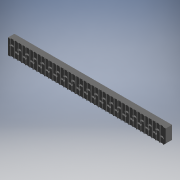
# Autodesk Inventor part: IDSD-20_ub
Saved by Autodesk Inventor 2017.3 (Build 213256000, 256)
## iProperties
Part Number: IDSD-20_ub
Material: Generic
Catalog Web Link: www.cadenas.de
Description: IDSS, IDSD Series - Upper Body-.100" Slim Body, IDC Ribbon Cable Assembly, Socket
Vendor: SAMTEC
Document SubType Name: Modeling
Designer: partserver
Manufacturer: SAMTEC
Mass: 0.43638 g
Surface Area: 11.6206 cm^2
Volume: 0.43638 cm^3
Density: 1 g/cm^3
Appearance: PSOLRGB-127-127-127
Category: PARTsolutions
Company: SAMTEC
Title: IDSD-20_ub
Author: Cadenas PARTsolutions
Comments: .100" Slim Body, IDC Ribbon Cable Assembly, Socket
PSOL_IDENT_0: {$CADENAS_DATA\23d-libs\samtec\modelling\idsd\parts\idsd_upper_body.prj},187 {VTYP=3D},{NB=IDSD-20_u
PSOL_IDENT_1: b},{LINA=IDSD-20_ub},{NN=IDSS, IDSD Series - Upper Body},{DATE=12.08.2019 09:04:52},{GEOMDATE=14.12.
PSOL_IDENT_2: 2015 10:21:00},{VERSION=},{LINEID=20},{WBVAR=POS},{WBNUMERIC=}  {NB=IDSD-20_ub},{LINA=IDSD-20_ub},{K
PSOL_IDENT_3: T=DUMMY},{PN=IDSD-20},{SERIES=IDSD},{POS=20},{POSNO=20},{A=2.05900000},{B=0.20},{C=0.10},{D=0.365}
NB: IDSD-20_ub
NN: IDSS, IDSD Series - Upper Body
NT: .100" Slim Body, IDC Ribbon Cable Assembly, Socket
NBSYN: $PN._ub
LINA: IDSD-20_ub
CATALOG: Samtec
SERIES: IDSD
POS: -20
B: 0.2
C: 0.1
SUPPLIER: SAMTEC
ARTICLENO: IDSD-20_ub
BOMINFO: IDSD-20_ub
CREATOR: CADENAS GmbH
Autodesk Inventor part; units mm, degrees
sketch "Sketch_1" plane through (0, 0, 0) normal (0, 1, 0) x (-1, 0, 0)
  line L0 (26.1493, 1.778) -> (25.3873, 2.54)
  line L1 (25.3873, 2.54) -> (-26.1493, 2.54)
  line L2 (-26.1493, 2.54) -> (-26.1493, -2.54)
  line L3 (-26.1493, -2.54) -> (26.1493, -2.54)
  line L4 (26.1493, -2.54) -> (26.1493, 1.778)
  line L5 (-24.2126, -0.9144) -> (-24.2126, -0.4064)
  line L6 (-24.2126, -0.4064) -> (-25.5461, -0.4064)
  line L7 (-25.5461, -0.4064) -> (-25.5461, -0.9144)
  line L8 (-25.5461, -0.9144) -> (-24.2126, -0.9144)
  line L9 (-22.714, 0.4064) -> (-22.714, 0.9144)
  line L10 (-22.714, 0.9144) -> (-24.0475, 0.9144)
  line L11 (-24.0475, 0.9144) -> (-24.0475, 0.4064)
  line L12 (-24.0475, 0.4064) -> (-22.714, 0.4064)
  line L13 (-21.6726, -0.9144) -> (-21.6726, -0.4064)
  line L14 (-21.6726, -0.4064) -> (-23.0061, -0.4064)
  line L15 (-23.0061, -0.4064) -> (-23.0061, -0.9144)
  line L16 (-23.0061, -0.9144) -> (-21.6726, -0.9144)
  line L17 (-20.174, 0.4064) -> (-20.174, 0.9144)
  line L18 (-20.174, 0.9144) -> (-21.5075, 0.9144)
  line L19 (-21.5075, 0.9144) -> (-21.5075, 0.4064)
  line L20 (-21.5075, 0.4064) -> (-20.174, 0.4064)
  line L21 (-19.1325, -0.9144) -> (-19.1325, -0.4064)
  line L22 (-19.1325, -0.4064) -> (-20.466, -0.4064)
  line L23 (-20.466, -0.4064) -> (-20.466, -0.9144)
  line L24 (-20.466, -0.9144) -> (-19.1325, -0.9144)
  line L25 (-17.6339, 0.4064) -> (-17.6339, 0.9144)
  line L26 (-17.6339, 0.9144) -> (-18.9674, 0.9144)
  line L27 (-18.9674, 0.9144) -> (-18.9674, 0.4064)
  line L28 (-18.9674, 0.4064) -> (-17.6339, 0.4064)
  line L29 (-16.5925, -0.9144) -> (-16.5925, -0.4064)
  line L30 (-16.5925, -0.4064) -> (-17.9261, -0.4064)
  line L31 (-17.9261, -0.4064) -> (-17.9261, -0.9144)
  line L32 (-17.9261, -0.9144) -> (-16.5925, -0.9144)
  line L33 (-15.0939, 0.4064) -> (-15.0939, 0.9144)
  line L34 (-15.0939, 0.9144) -> (-16.4275, 0.9144)
  line L35 (-16.4275, 0.9144) -> (-16.4275, 0.4064)
  line L36 (-16.4275, 0.4064) -> (-15.0939, 0.4064)
  line L37 (-14.0526, -0.9144) -> (-14.0526, -0.4064)
  line L38 (-14.0526, -0.4064) -> (-15.3861, -0.4064)
  line L39 (-15.3861, -0.4064) -> (-15.3861, -0.9144)
  line L40 (-15.3861, -0.9144) -> (-14.0526, -0.9144)
  line L41 (-12.554, 0.4064) -> (-12.554, 0.9144)
  line L42 (-12.554, 0.9144) -> (-13.8874, 0.9144)
  line L43 (-13.8874, 0.9144) -> (-13.8874, 0.4064)
  line L44 (-13.8874, 0.4064) -> (-12.554, 0.4064)
  line L45 (-11.5125, -0.9144) -> (-11.5125, -0.4064)
  line L46 (-11.5125, -0.4064) -> (-12.846, -0.4064)
  line L47 (-12.846, -0.4064) -> (-12.846, -0.9144)
  line L48 (-12.846, -0.9144) -> (-11.5125, -0.9144)
  line L49 (-10.014, 0.4064) -> (-10.014, 0.9144)
  line L50 (-10.014, 0.9144) -> (-11.3474, 0.9144)
  line L51 (-11.3474, 0.9144) -> (-11.3474, 0.4064)
  line L52 (-11.3474, 0.4064) -> (-10.014, 0.4064)
  line L53 (-8.9726, -0.9144) -> (-8.9726, -0.4064)
  line L54 (-8.9726, -0.4064) -> (-10.306, -0.4064)
  line L55 (-10.306, -0.4064) -> (-10.306, -0.9144)
  line L56 (-10.306, -0.9144) -> (-8.9726, -0.9144)
  line L57 (-7.474, 0.4064) -> (-7.474, 0.9144)
  line L58 (-7.474, 0.9144) -> (-8.8074, 0.9144)
  line L59 (-8.8074, 0.9144) -> (-8.8074, 0.4064)
  line L60 (-8.8074, 0.4064) -> (-7.474, 0.4064)
  line L61 (-6.4325, -0.9144) -> (-6.4325, -0.4064)
  line L62 (-6.4325, -0.4064) -> (-7.7661, -0.4064)
  line L63 (-7.7661, -0.4064) -> (-7.7661, -0.9144)
  line L64 (-7.7661, -0.9144) -> (-6.4325, -0.9144)
  line L65 (-4.934, 0.4064) -> (-4.934, 0.9144)
  line L66 (-4.934, 0.9144) -> (-6.2675, 0.9144)
  line L67 (-6.2675, 0.9144) -> (-6.2675, 0.4064)
  line L68 (-6.2675, 0.4064) -> (-4.934, 0.4064)
  line L69 (-3.8925, -0.9144) -> (-3.8925, -0.4064)
  line L70 (-3.8925, -0.4064) -> (-5.226, -0.4064)
  line L71 (-5.226, -0.4064) -> (-5.226, -0.9144)
  line L72 (-5.226, -0.9144) -> (-3.8925, -0.9144)
  line L73 (-2.3939, 0.4064) -> (-2.3939, 0.9144)
  line L74 (-2.3939, 0.9144) -> (-3.7275, 0.9144)
  line L75 (-3.7275, 0.9144) -> (-3.7275, 0.4064)
  line L76 (-3.7275, 0.4064) -> (-2.3939, 0.4064)
  line L77 (-1.3525, -0.9144) -> (-1.3525, -0.4064)
  line L78 (-1.3525, -0.4064) -> (-2.686, -0.4064)
  line L79 (-2.686, -0.4064) -> (-2.686, -0.9144)
  line L80 (-2.686, -0.9144) -> (-1.3525, -0.9144)
  line L81 (0.1461, 0.4064) -> (0.1461, 0.9144)
  line L82 (0.1461, 0.9144) -> (-1.1875, 0.9144)
  line L83 (-1.1875, 0.9144) -> (-1.1875, 0.4064)
  line L84 (-1.1875, 0.4064) -> (0.1461, 0.4064)
  line L85 (1.1875, -0.9144) -> (1.1875, -0.4064)
  line L86 (1.1875, -0.4064) -> (-0.146, -0.4064)
  line L87 (-0.146, -0.4064) -> (-0.146, -0.9144)
  line L88 (-0.146, -0.9144) -> (1.1875, -0.9144)
  line L89 (2.686, 0.4064) -> (2.686, 0.9144)
  line L90 (2.686, 0.9144) -> (1.3525, 0.9144)
  line L91 (1.3525, 0.9144) -> (1.3525, 0.4064)
  line L92 (1.3525, 0.4064) -> (2.686, 0.4064)
  line L93 (3.7275, -0.9144) -> (3.7275, -0.4064)
  line L94 (3.7275, -0.4064) -> (2.3939, -0.4064)
  line L95 (2.3939, -0.4064) -> (2.3939, -0.9144)
  line L96 (2.3939, -0.9144) -> (3.7275, -0.9144)
  line L97 (5.226, 0.4064) -> (5.226, 0.9144)
  line L98 (5.226, 0.9144) -> (3.8925, 0.9144)
  line L99 (3.8925, 0.9144) -> (3.8925, 0.4064)
  line L100 (3.8925, 0.4064) -> (5.226, 0.4064)
  line L101 (6.2675, -0.9144) -> (6.2675, -0.4064)
  line L102 (6.2675, -0.4064) -> (4.934, -0.4064)
  line L103 (4.934, -0.4064) -> (4.934, -0.9144)
  line L104 (4.934, -0.9144) -> (6.2675, -0.9144)
  line L105 (7.7661, 0.4064) -> (7.7661, 0.9144)
  line L106 (7.7661, 0.9144) -> (6.4325, 0.9144)
  line L107 (6.4325, 0.9144) -> (6.4325, 0.4064)
  line L108 (6.4325, 0.4064) -> (7.7661, 0.4064)
  line L109 (8.8074, -0.9144) -> (8.8074, -0.4064)
  line L110 (8.8074, -0.4064) -> (7.474, -0.4064)
  line L111 (7.474, -0.4064) -> (7.474, -0.9144)
  line L112 (7.474, -0.9144) -> (8.8074, -0.9144)
  line L113 (10.306, 0.4064) -> (10.306, 0.9144)
  line L114 (10.306, 0.9144) -> (8.9726, 0.9144)
  line L115 (8.9726, 0.9144) -> (8.9726, 0.4064)
  line L116 (8.9726, 0.4064) -> (10.306, 0.4064)
  line L117 (11.3474, -0.9144) -> (11.3474, -0.4064)
  line L118 (11.3474, -0.4064) -> (10.014, -0.4064)
  line L119 (10.014, -0.4064) -> (10.014, -0.9144)
  line L120 (10.014, -0.9144) -> (11.3474, -0.9144)
  line L121 (12.846, 0.4064) -> (12.846, 0.9144)
  line L122 (12.846, 0.9144) -> (11.5125, 0.9144)
  line L123 (11.5125, 0.9144) -> (11.5125, 0.4064)
  line L124 (11.5125, 0.4064) -> (12.846, 0.4064)
  line L125 (13.8874, -0.9144) -> (13.8874, -0.4064)
  line L126 (13.8874, -0.4064) -> (12.554, -0.4064)
  line L127 (12.554, -0.4064) -> (12.554, -0.9144)
  line L128 (12.554, -0.9144) -> (13.8874, -0.9144)
  line L129 (15.3861, 0.4064) -> (15.3861, 0.9144)
  line L130 (15.3861, 0.9144) -> (14.0526, 0.9144)
  line L131 (14.0526, 0.9144) -> (14.0526, 0.4064)
  line L132 (14.0526, 0.4064) -> (15.3861, 0.4064)
  line L133 (16.4275, -0.9144) -> (16.4275, -0.4064)
  line L134 (16.4275, -0.4064) -> (15.0939, -0.4064)
  line L135 (15.0939, -0.4064) -> (15.0939, -0.9144)
  line L136 (15.0939, -0.9144) -> (16.4275, -0.9144)
  line L137 (17.9261, 0.4064) -> (17.9261, 0.9144)
  line L138 (17.9261, 0.9144) -> (16.5925, 0.9144)
  line L139 (16.5925, 0.9144) -> (16.5925, 0.4064)
  line L140 (16.5925, 0.4064) -> (17.9261, 0.4064)
  line L141 (18.9674, -0.9144) -> (18.9674, -0.4064)
  line L142 (18.9674, -0.4064) -> (17.6339, -0.4064)
  line L143 (17.6339, -0.4064) -> (17.6339, -0.9144)
  line L144 (17.6339, -0.9144) -> (18.9674, -0.9144)
  line L145 (20.466, 0.4064) -> (20.466, 0.9144)
  line L146 (20.466, 0.9144) -> (19.1325, 0.9144)
  line L147 (19.1325, 0.9144) -> (19.1325, 0.4064)
  line L148 (19.1325, 0.4064) -> (20.466, 0.4064)
  line L149 (21.5075, -0.9144) -> (21.5075, -0.4064)
  line L150 (21.5075, -0.4064) -> (20.174, -0.4064)
  line L151 (20.174, -0.4064) -> (20.174, -0.9144)
  line L152 (20.174, -0.9144) -> (21.5075, -0.9144)
  line L153 (23.0061, 0.4064) -> (23.0061, 0.9144)
  line L154 (23.0061, 0.9144) -> (21.6726, 0.9144)
  line L155 (21.6726, 0.9144) -> (21.6726, 0.4064)
  line L156 (21.6726, 0.4064) -> (23.0061, 0.4064)
  line L157 (24.0475, -0.9144) -> (24.0475, -0.4064)
  line L158 (24.0475, -0.4064) -> (22.714, -0.4064)
  line L159 (22.714, -0.4064) -> (22.714, -0.9144)
  line L160 (22.714, -0.9144) -> (24.0475, -0.9144)
  line L161 (25.5461, 0.4064) -> (25.5461, 0.9144)
  line L162 (25.5461, 0.9144) -> (24.2126, 0.9144)
  line L163 (24.2126, 0.9144) -> (24.2126, 0.4064)
  line L164 (24.2126, 0.4064) -> (25.5461, 0.4064)
  constraints: 330 end point
extrude "Extrusion1" add sketch "Sketch_1" along normal blind 2.286
sketch "Sketch_7" plane through (0, 0, 0) normal (0, 0, 1) x (1, 0, 0)
  line L0 (-27.4193, -1.27) -> (27.4193, -1.27)
  line L1 (27.4193, -1.27) -> (27.4193, 1.27)
  line L2 (27.4193, 1.27) -> (26.1493, 1.27)
  line L3 (26.1493, 1.27) -> (26.1493, 0.1524)
  line L4 (26.1493, 0.1524) -> (25.5143, 0.1524)
  arc A0 (25.3365, 0.3302) -> (25.5143, 0.1524) centre (25.5143, 0.3302) ccw
  line L5 (25.3365, 0.3302) -> (25.3365, 0.4064)
  line L6 (25.3365, 0.4064) -> (24.4221, 0.4064)
  line L7 (24.4221, 0.4064) -> (24.4221, 0.3302)
  arc A1 (24.0665, 0.3302) -> (24.4221, 0.3302) centre (24.2443, 0.3302) ccw
  line L8 (24.0665, 0.3302) -> (24.0665, 0.4064)
  line L9 (24.0665, 0.4064) -> (23.1521, 0.4064)
  line L10 (23.1521, 0.4064) -> (23.1521, 0.3302)
  arc A2 (22.7965, 0.3302) -> (23.1521, 0.3302) centre (22.9743, 0.3302) ccw
  line L11 (22.7965, 0.3302) -> (22.7965, 0.4064)
  line L12 (22.7965, 0.4064) -> (21.8821, 0.4064)
  line L13 (21.8821, 0.4064) -> (21.8821, 0.3302)
  arc A3 (21.5265, 0.3302) -> (21.8821, 0.3302) centre (21.7043, 0.3302) ccw
  line L14 (21.5265, 0.3302) -> (21.5265, 0.4064)
  line L15 (21.5265, 0.4064) -> (20.6121, 0.4064)
  line L16 (20.6121, 0.4064) -> (20.6121, 0.3302)
  arc A4 (20.2565, 0.3302) -> (20.6121, 0.3302) centre (20.4343, 0.3302) ccw
  line L17 (20.2565, 0.3302) -> (20.2565, 0.4064)
  line L18 (20.2565, 0.4064) -> (19.3421, 0.4064)
  line L19 (19.3421, 0.4064) -> (19.3421, 0.3302)
  arc A5 (18.9865, 0.3302) -> (19.3421, 0.3302) centre (19.1643, 0.3302) ccw
  line L20 (18.9865, 0.3302) -> (18.9865, 0.4064)
  line L21 (18.9865, 0.4064) -> (18.0721, 0.4064)
  line L22 (18.0721, 0.4064) -> (18.0721, 0.3302)
  arc A6 (17.7165, 0.3302) -> (18.0721, 0.3302) centre (17.8943, 0.3302) ccw
  line L23 (17.7165, 0.3302) -> (17.7165, 0.4064)
  line L24 (17.7165, 0.4064) -> (16.8021, 0.4064)
  line L25 (16.8021, 0.4064) -> (16.8021, 0.3302)
  arc A7 (16.4465, 0.3302) -> (16.8021, 0.3302) centre (16.6243, 0.3302) ccw
  line L26 (16.4465, 0.3302) -> (16.4465, 0.4064)
  line L27 (16.4465, 0.4064) -> (15.5321, 0.4064)
  line L28 (15.5321, 0.4064) -> (15.5321, 0.3302)
  arc A8 (15.1765, 0.3302) -> (15.5321, 0.3302) centre (15.3543, 0.3302) ccw
  line L29 (15.1765, 0.3302) -> (15.1765, 0.4064)
  line L30 (15.1765, 0.4064) -> (14.2621, 0.4064)
  line L31 (14.2621, 0.4064) -> (14.2621, 0.3302)
  arc A9 (13.9065, 0.3302) -> (14.2621, 0.3302) centre (14.0843, 0.3302) ccw
  line L32 (13.9065, 0.3302) -> (13.9065, 0.4064)
  line L33 (13.9065, 0.4064) -> (12.9921, 0.4064)
  line L34 (12.9921, 0.4064) -> (12.9921, 0.3302)
  arc A10 (12.6365, 0.3302) -> (12.9921, 0.3302) centre (12.8143, 0.3302) ccw
  line L35 (12.6365, 0.3302) -> (12.6365, 0.4064)
  line L36 (12.6365, 0.4064) -> (11.7221, 0.4064)
  line L37 (11.7221, 0.4064) -> (11.7221, 0.3302)
  arc A11 (11.3665, 0.3302) -> (11.7221, 0.3302) centre (11.5443, 0.3302) ccw
  line L38 (11.3665, 0.3302) -> (11.3665, 0.4064)
  line L39 (11.3665, 0.4064) -> (10.4521, 0.4064)
  line L40 (10.4521, 0.4064) -> (10.4521, 0.3302)
  arc A12 (10.0965, 0.3302) -> (10.4521, 0.3302) centre (10.2743, 0.3302) ccw
  line L41 (10.0965, 0.3302) -> (10.0965, 0.4064)
  line L42 (10.0965, 0.4064) -> (9.1821, 0.4064)
  line L43 (9.1821, 0.4064) -> (9.1821, 0.3302)
  arc A13 (8.8265, 0.3302) -> (9.1821, 0.3302) centre (9.0043, 0.3302) ccw
  line L44 (8.8265, 0.3302) -> (8.8265, 0.4064)
  line L45 (8.8265, 0.4064) -> (7.9121, 0.4064)
  line L46 (7.9121, 0.4064) -> (7.9121, 0.3302)
  arc A14 (7.5565, 0.3302) -> (7.9121, 0.3302) centre (7.7343, 0.3302) ccw
  line L47 (7.5565, 0.3302) -> (7.5565, 0.4064)
  line L48 (7.5565, 0.4064) -> (6.6421, 0.4064)
  line L49 (6.6421, 0.4064) -> (6.6421, 0.3302)
  arc A15 (6.2865, 0.3302) -> (6.6421, 0.3302) centre (6.4643, 0.3302) ccw
  line L50 (6.2865, 0.3302) -> (6.2865, 0.4064)
  line L51 (6.2865, 0.4064) -> (5.3721, 0.4064)
  line L52 (5.3721, 0.4064) -> (5.3721, 0.3302)
  arc A16 (5.0165, 0.3302) -> (5.3721, 0.3302) centre (5.1943, 0.3302) ccw
  line L53 (5.0165, 0.3302) -> (5.0165, 0.4064)
  line L54 (5.0165, 0.4064) -> (4.1021, 0.4064)
  line L55 (4.1021, 0.4064) -> (4.1021, 0.3302)
  arc A17 (3.7465, 0.3302) -> (4.1021, 0.3302) centre (3.9243, 0.3302) ccw
  line L56 (3.7465, 0.3302) -> (3.7465, 0.4064)
  line L57 (3.7465, 0.4064) -> (2.8321, 0.4064)
  line L58 (2.8321, 0.4064) -> (2.8321, 0.3302)
  arc A18 (2.4765, 0.3302) -> (2.8321, 0.3302) centre (2.6543, 0.3302) ccw
  line L59 (2.4765, 0.3302) -> (2.4765, 0.4064)
  line L60 (2.4765, 0.4064) -> (1.5621, 0.4064)
  line L61 (1.5621, 0.4064) -> (1.5621, 0.3302)
  arc A19 (1.2065, 0.3302) -> (1.5621, 0.3302) centre (1.3843, 0.3302) ccw
  line L62 (1.2065, 0.3302) -> (1.2065, 0.4064)
  line L63 (1.2065, 0.4064) -> (0.2921, 0.4064)
  line L64 (0.2921, 0.4064) -> (0.2921, 0.3302)
  arc A20 (-0.0635, 0.3302) -> (0.2921, 0.3302) centre (0.1143, 0.3302) ccw
  line L65 (-0.0635, 0.3302) -> (-0.0635, 0.4064)
  line L66 (-0.0635, 0.4064) -> (-0.9779, 0.4064)
  line L67 (-0.9779, 0.4064) -> (-0.9779, 0.3302)
  arc A21 (-1.3335, 0.3302) -> (-0.9779, 0.3302) centre (-1.1557, 0.3302) ccw
  line L68 (-1.3335, 0.3302) -> (-1.3335, 0.4064)
  line L69 (-1.3335, 0.4064) -> (-2.2479, 0.4064)
  line L70 (-2.2479, 0.4064) -> (-2.2479, 0.3302)
  arc A22 (-2.6035, 0.3302) -> (-2.2479, 0.3302) centre (-2.4257, 0.3302) ccw
  line L71 (-2.6035, 0.3302) -> (-2.6035, 0.4064)
  line L72 (-2.6035, 0.4064) -> (-3.5179, 0.4064)
  line L73 (-3.5179, 0.4064) -> (-3.5179, 0.3302)
  arc A23 (-3.8735, 0.3302) -> (-3.5179, 0.3302) centre (-3.6957, 0.3302) ccw
  line L74 (-3.8735, 0.3302) -> (-3.8735, 0.4064)
  line L75 (-3.8735, 0.4064) -> (-4.7879, 0.4064)
  line L76 (-4.7879, 0.4064) -> (-4.7879, 0.3302)
  arc A24 (-5.1435, 0.3302) -> (-4.7879, 0.3302) centre (-4.9657, 0.3302) ccw
  line L77 (-5.1435, 0.3302) -> (-5.1435, 0.4064)
  line L78 (-5.1435, 0.4064) -> (-6.0579, 0.4064)
  line L79 (-6.0579, 0.4064) -> (-6.0579, 0.3302)
  arc A25 (-6.4135, 0.3302) -> (-6.0579, 0.3302) centre (-6.2357, 0.3302) ccw
  line L80 (-6.4135, 0.3302) -> (-6.4135, 0.4064)
  line L81 (-6.4135, 0.4064) -> (-7.3279, 0.4064)
  line L82 (-7.3279, 0.4064) -> (-7.3279, 0.3302)
  arc A26 (-7.6835, 0.3302) -> (-7.3279, 0.3302) centre (-7.5057, 0.3302) ccw
  line L83 (-7.6835, 0.3302) -> (-7.6835, 0.4064)
  line L84 (-7.6835, 0.4064) -> (-8.5979, 0.4064)
  line L85 (-8.5979, 0.4064) -> (-8.5979, 0.3302)
  arc A27 (-8.9535, 0.3302) -> (-8.5979, 0.3302) centre (-8.7757, 0.3302) ccw
  line L86 (-8.9535, 0.3302) -> (-8.9535, 0.4064)
  line L87 (-8.9535, 0.4064) -> (-9.8679, 0.4064)
  line L88 (-9.8679, 0.4064) -> (-9.8679, 0.3302)
  arc A28 (-10.2235, 0.3302) -> (-9.8679, 0.3302) centre (-10.0457, 0.3302) ccw
  line L89 (-10.2235, 0.3302) -> (-10.2235, 0.4064)
  line L90 (-10.2235, 0.4064) -> (-11.1379, 0.4064)
  line L91 (-11.1379, 0.4064) -> (-11.1379, 0.3302)
  arc A29 (-11.4935, 0.3302) -> (-11.1379, 0.3302) centre (-11.3157, 0.3302) ccw
  line L92 (-11.4935, 0.3302) -> (-11.4935, 0.4064)
  line L93 (-11.4935, 0.4064) -> (-12.4079, 0.4064)
  line L94 (-12.4079, 0.4064) -> (-12.4079, 0.3302)
  arc A30 (-12.7635, 0.3302) -> (-12.4079, 0.3302) centre (-12.5857, 0.3302) ccw
  line L95 (-12.7635, 0.3302) -> (-12.7635, 0.4064)
  line L96 (-12.7635, 0.4064) -> (-13.6779, 0.4064)
  line L97 (-13.6779, 0.4064) -> (-13.6779, 0.3302)
  arc A31 (-14.0335, 0.3302) -> (-13.6779, 0.3302) centre (-13.8557, 0.3302) ccw
  line L98 (-14.0335, 0.3302) -> (-14.0335, 0.4064)
  line L99 (-14.0335, 0.4064) -> (-14.9479, 0.4064)
  line L100 (-14.9479, 0.4064) -> (-14.9479, 0.3302)
  arc A32 (-15.3035, 0.3302) -> (-14.9479, 0.3302) centre (-15.1257, 0.3302) ccw
  line L101 (-15.3035, 0.3302) -> (-15.3035, 0.4064)
  line L102 (-15.3035, 0.4064) -> (-16.2179, 0.4064)
  line L103 (-16.2179, 0.4064) -> (-16.2179, 0.3302)
  arc A33 (-16.5735, 0.3302) -> (-16.2179, 0.3302) centre (-16.3957, 0.3302) ccw
  line L104 (-16.5735, 0.3302) -> (-16.5735, 0.4064)
  line L105 (-16.5735, 0.4064) -> (-17.4879, 0.4064)
  line L106 (-17.4879, 0.4064) -> (-17.4879, 0.3302)
  arc A34 (-17.8435, 0.3302) -> (-17.4879, 0.3302) centre (-17.6657, 0.3302) ccw
  line L107 (-17.8435, 0.3302) -> (-17.8435, 0.4064)
  line L108 (-17.8435, 0.4064) -> (-18.7579, 0.4064)
  line L109 (-18.7579, 0.4064) -> (-18.7579, 0.3302)
  arc A35 (-19.1135, 0.3302) -> (-18.7579, 0.3302) centre (-18.9357, 0.3302) ccw
  line L110 (-19.1135, 0.3302) -> (-19.1135, 0.4064)
  line L111 (-19.1135, 0.4064) -> (-20.0279, 0.4064)
  line L112 (-20.0279, 0.4064) -> (-20.0279, 0.3302)
  arc A36 (-20.3835, 0.3302) -> (-20.0279, 0.3302) centre (-20.2057, 0.3302) ccw
  line L113 (-20.3835, 0.3302) -> (-20.3835, 0.4064)
  line L114 (-20.3835, 0.4064) -> (-21.2979, 0.4064)
  line L115 (-21.2979, 0.4064) -> (-21.2979, 0.3302)
  arc A37 (-21.6535, 0.3302) -> (-21.2979, 0.3302) centre (-21.4757, 0.3302) ccw
  line L116 (-21.6535, 0.3302) -> (-21.6535, 0.4064)
  line L117 (-21.6535, 0.4064) -> (-22.5679, 0.4064)
  line L118 (-22.5679, 0.4064) -> (-22.5679, 0.3302)
  arc A38 (-22.9235, 0.3302) -> (-22.5679, 0.3302) centre (-22.7457, 0.3302) ccw
  line L119 (-22.9235, 0.3302) -> (-22.9235, 0.4064)
  line L120 (-22.9235, 0.4064) -> (-23.8379, 0.4064)
  line L121 (-23.8379, 0.4064) -> (-23.8379, 0.3302)
  arc A39 (-24.1935, 0.3302) -> (-23.8379, 0.3302) centre (-24.0157, 0.3302) ccw
  line L122 (-24.1935, 0.3302) -> (-24.1935, 0.4064)
  line L123 (-24.1935, 0.4064) -> (-25.1079, 0.4064)
  line L124 (-25.1079, 0.4064) -> (-25.1079, 0.3302)
  arc A40 (-25.2857, 0.1524) -> (-25.1079, 0.3302) centre (-25.2857, 0.3302) ccw
  line L125 (-25.2857, 0.1524) -> (-26.1493, 0.1524)
  line L126 (-26.1493, 0.1524) -> (-26.1493, 1.27)
  line L127 (-26.1493, 1.27) -> (-27.4193, 1.27)
  line L128 (-27.4193, 1.27) -> (-27.4193, -1.27)
  constraints: 258 end point, 82 point on circle, 41 centre point
extrude "Extrusion2" cut sketch "Sketch_7" along normal mid plane 5.08
sketch "Sketch_12" plane through (0, 2.286, 0) normal (0, 1, 0) x (1, 0, 0)
  line L0 (-24.4729, 0.9144) -> (-24.4729, 0.4064)
  line L1 (-24.4729, 0.4064) -> (-22.2885, 0.4064)
  line L2 (-22.2885, 0.4064) -> (-22.2885, 0.9144)
  line L3 (-22.2885, 0.9144) -> (-24.4729, 0.9144)
  constraints: 8 end point
extrude "Extrusion3" cut sketch "Sketch_12" against normal blind 1.5748
pattern_linear "Rectangular Pattern1" count 20 spacing 2.54 along (1, 0, 0) of "Extrusion3"
sketch "Sketch_14" plane through (0, 2.286, 0) normal (0, 1, 0) x (1, 0, 0)
  line L0 (-25.9715, -0.4064) -> (-25.9715, -0.9144)
  line L1 (-25.9715, -0.9144) -> (-23.7871, -0.9144)
  line L2 (-23.7871, -0.9144) -> (-23.7871, -0.4064)
  line L3 (-23.7871, -0.4064) -> (-25.9715, -0.4064)
  constraints: 8 end point
extrude "Extrusion4" cut sketch "Sketch_14" against normal blind 1.5748
pattern_linear "Rectangular Pattern2" count 20 spacing 2.54 along (1, 0, 0) of "Extrusion4"
ref_plane "upper_body_to_lower_body_XY" through (0, 2.286, 0) normal (0, 1, 0) x (1, 0, 0)
ref_plane "upper_body_to_lower_body_YZ" through (0, 2.286, 0) normal (1, 0, 0) x (0, 0, -1)
ref_plane "upper_body_to_lower_body_ZX" through (0, 2.286, 0) normal (0, 0, -1) x (0, 1, 0)
ref_plane "upper_body_to_lower_body_reverse_XY" through (0, 2.286, 0) normal (0, -1, 0) x (1, 0, 0)
ref_plane "upper_body_to_lower_body_reverse_YZ" through (0, 2.286, 0) normal (1, 0, 0) x (0, 0, 1)
ref_plane "upper_body_to_lower_body_reverse_ZX" through (0, 2.286, 0) normal (0, 0, 1) x (0, -1, 0)
body "Solid1"
